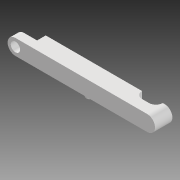
# Autodesk Inventor part: RegulatorHinge
Saved by Autodesk Inventor 2020 (Build 240168000, 168)
## iProperties
Created: 2021-05-21
Part Number: RegulatorHinge
Material: Generic
Document SubType Name: Modeling
Designer: DDeGo
Density: 1 g/cm^3
Appearance: Default
Author: DDeGo
Autodesk Inventor part; units mm, degrees
ref_plane "YZ Plane" through (0, 0, 0) normal (1, 0, 0) x (0, 1, 0)
ref_plane "XZ Plane" through (0, 0, 0) normal (0, 1, 0) x (-1, 0, 0)
ref_plane "XY Plane" through (0, 0, 0) normal (0, 0, 1) x (1, 0, 0)
sketch "Sketch1" plane through (0, 0, 0) normal (0, 0, 1) x (1, 0, 0)
  line L0 (-19, 0) -> (19, 0) construction
  line L1 (-19, -2.25) -> (19, -2.25)
  line L2 (19, 2.25) -> (-19, 2.25)
  arc A0 (-19, 2.25) -> (-19, -2.25) centre (-19, 0) ccw
  arc A1 (19, -2.25) -> (19, 2.25) centre (19, 0) ccw
  circle A2 centre (-19, 0) radius 1.35
  point P0 (0, 0)
  dimension "d0" = 4.5
  dimension "d1" = 38
  dimension "d8" = 2.7
  constraints: 8 end point, 4 point on circle, 4 tangent, 3 centre point, 1 coincident, 1 horizontal, 1 midpoint, 1 parallel
  measures "d0" distance between parallel lines of L1 L2
  measures "d1" distance of L0.start L0.end
  measures "d8" diameter of A2
extrude "Extrusion1" add sketch "Sketch1" along normal mid plane 10
sketch "Sketch2" plane through (-19, 2.25, -5) normal (0, 1, 0) x (1, 0, 0)
  line L0 (-8.25, -7.5) -> (3.75, -7.5)
  line L1 (3.75, -7.5) -> (3.75, -2.5)
  line L2 (3.75, -2.5) -> (-8.25, -2.5)
  line L3 (-8.25, -2.5) -> (-8.25, -7.5)
  line L4 (-2.25, 0) -> (-2.25, -10) projected
  line L5 (-8.25, -7.5) -> (3.75, -2.5) construction
  line L6 (3.75, -7.5) -> (-8.25, -2.5) construction
  point P0 (19, -5)
  point P1 (-2.25, -5)
  dimension "d4" = 5
  dimension "d5" = 6
  constraints: 12 end point, 3 midpoint, 2 parallel, 1 horizontal, 1 perpendicular
  measures "d4" distance between parallel lines of L0 L2
  measures "d5" distance between parallel lines of L4 L1
extrude "Extrusion2" cut sketch "Sketch2" against normal through all
sketch "Sketch3" plane through (-19, 2.25, -5) normal (0, 1, 0) x (1, 0, 0)
  line L0 (1.35, -10) -> (-1.35, -10) construction
  line L1 (-1.35, 0) -> (1.35, 0) construction
  line L2 (0, -7.5) -> (0, -10) construction
  line L3 (0, -10) -> (0, 0) construction
  line L4 (0, -5) -> (34.5, -5) construction
  line L5 (35.5, -5) -> (33.5, -5) construction
  line L6 (35.5, -3) -> (33.5, -3)
  line L7 (33.5, -7) -> (35.5, -7)
  arc A0 (35.5, -7) -> (35.5, -3) centre (35.5, -5) ccw
  arc A1 (33.5, -3) -> (33.5, -7) centre (33.5, -5) ccw
  point P0 (19, -5)
  dimension "d9" = 34.5
  dimension "d11" = 2
  dimension "d12" = 2
  constraints: 12 end point, 4 point on circle, 4 tangent, 3 midpoint, 2 centre point, 1 horizontal, 1 parallel, 1 point on line
  measures "d9" distance of L4.start L4.end
  measures "d11" radius of A1
  measures "d12" distance of L6.start L6.end
extrude "Extrusion3" cut sketch "Sketch3" against normal through all
sketch "Sketch4" plane through (0, 0, 0) normal (0, 0, 1) x (1, 0, 0)
  line L0 (-19, -2.25) -> (19, -2.25) projected
  line L1 (-2.75, -2.25) -> (-2.75, -7.25)
  line L2 (-3.6897, -6.592) -> (-5.2701, -2.25)
  arc A0 (-3.6897, -6.592) -> (-2.75, -7.25) centre (-2.75, -6.25) ccw
  circle A1 centre (-19, 0) radius 1.35 projected
  point P0 (0, 0)
  dimension "d15" = 1
  dimension "d16" = 70
  dimension "d18" = 16.25
  dimension "d21" = 5
  constraints: 4 end point, 3 point on line, 2 point on circle, 1 centre point, 1 tangent, 1 vertical
  measures "d15" radius of A0
  measures "d16" angle of L0 L2
  measures "d18" distance from line of A1.centre L1
  measures "d21" distance of L1.start L1.end
revolve "Revolution1" add sketch "Sketch4" angle 360 about axis through (-2.75, -2.25, 0) along (0, -1, 0) contours L0 L1 A0 L2
sketch "Sketch5" plane through (-19, 2.25, 5) normal (0, 1, 0) x (1, 0, 0)
  line L0 (42.5072, 5) -> (-11.8612, 5)
  line L1 (-11.8612, 5) -> (-11.8612, 14.1834)
  line L2 (-11.8612, 14.1834) -> (42.5072, 14.1834)
  line L3 (42.5072, 14.1834) -> (42.5072, 5)
  point P0 (19, 5)
  constraints: 8 end point, 2 parallel, 1 horizontal, 1 perpendicular, 1 point on line
extrude "Extrusion4" cut sketch "Sketch5" against normal through all
body "Solid1"
